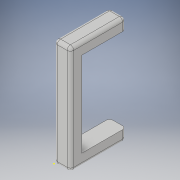
# Autodesk Inventor part: Bumper
Saved by Autodesk Inventor 2018 (Build 220112000, 112)
## iProperties
Created: 2018-01-19
Part Number: Bumper
Material: Generic
Document SubType Name: Modeling
Designer: s-4000369
Density: 1 g/cm^3
Appearance: Default
Author: s-4000369
Autodesk Inventor part; units mm, degrees
ref_plane "YZ Plane" through (0, 0, 0) normal (1, 0, 0) x (0, 1, 0)
ref_plane "XZ Plane" through (0, 0, 0) normal (0, 1, 0) x (-1, 0, 0)
ref_plane "XY Plane" through (0, 0, 0) normal (0, 0, 1) x (1, 0, 0)
sketch "Sketch1" plane through (0, 0, 0) normal (1, 0, 0) x (0, 1, 0)
  point P0 (0, 0)
sketch "Sketch2" plane through (0, 0, 0) normal (1, 0, 0) x (0, 1, 0)
  line L0 (0, 0) -> (0, -431.8)
  line L1 (0, -431.8) -> (88.9, -431.8)
  line L2 (88.9, -431.8) -> (88.9, -88.9)
  line L3 (88.9, -88.9) -> (749.3, -88.9)
  line L4 (749.3, -88.9) -> (749.3, -431.8)
  line L5 (749.3, -431.8) -> (838.2, -431.8)
  line L6 (838.2, -431.8) -> (838.2, 0)
  line L7 (838.2, 0) -> (0, 0)
  dimension "d0" = 660.4
  dimension "d1" = 342.9
  dimension "d2" = 342.9
  dimension "d3" = 88.9
  dimension "d4" = 88.9
  dimension "d5" = 88.9
  constraints: 16 end point, 6 perpendicular, 2 vertical
  measures "d0" distance of L2.end L3.end
  measures "d1" distance of L1.end L2.end
  measures "d2" distance of L3.end L4.end
  measures "d3" distance between parallel lines of L7 L3
  measures "d4" distance between parallel lines of L0 L2
  measures "d5" distance between parallel lines of L4 L6
extrude "Extrusion1" add sketch "Sketch2" along normal blind 127
fillet "Fillet1" radius 25.4 14 edges at (127, 419.1, 0) (0, 419.1, 0) (63.5, 838.2, 0) (127, 838.2, -215.9) (0, 838.2, -215.9) (63.5, 0, 0) (127, 0, -215.9) (127, 44.45, -431.8) (127, 793.75, -431.8) (63.5, 838.2, -431.8) (0, 793.75, -431.8) (0, 0, -215.9) (0, 44.45, -431.8) (63.5, 0, -431.8)
sketch "Sketch7" plane through (0, 88.9, -88.9) normal (0, 0, -1) x (-1, 0, 0)
  line L0 (-127, 0) -> (-127, 660.4) projected
  line L1 (-127, 0) -> (-127, 660.4)
  line L2 (-127, 660.4) -> (-127, 647.7)
  line L3 (-127, -63.5) -> (-127, 723.9) projected
  line L4 (-127, 0) -> (-127, 12.7)
  line L5 (-127, 12.7) -> (-127, 139.7)
  line L6 (-127, 139.7) -> (-127, 266.7)
  line L7 (-127, 266.7) -> (-127, 393.7)
  line L8 (-127, 393.7) -> (-127, 520.7)
  line L9 (-127, 520.7) -> (-127, 647.7)
  line L10 (-127, 330.2) -> (0, 330.2)
  line L11 (-127, 520.7) -> (0, 520.7)
  line L12 (0, 0) -> (0, 660.4) projected
  line L13 (-127, 139.7) -> (0, 139.7)
  line L14 (-127, 139.7) -> (-117.475, 139.7)
  line L15 (-127, 330.2) -> (-117.475, 330.2)
  line L16 (-127, 520.7) -> (-117.475, 520.7)
  line L17 (-117.475, 139.7) -> (-117.475, 165.1)
  line L18 (-117.475, 139.7) -> (-117.475, 114.3)
  line L19 (-117.475, 330.2) -> (-117.475, 304.8)
  line L20 (-117.475, 304.8) -> (-117.475, 355.6)
  line L21 (-117.475, 520.7) -> (-117.475, 495.3)
  line L22 (-117.475, 495.3) -> (-117.475, 546.1)
  circle A0 centre (-117.475, 114.3) radius 2.54
  circle A1 centre (-117.475, 165.1) radius 2.54
  circle A2 centre (-117.475, 304.8) radius 2.54
  circle A3 centre (-117.475, 355.6) radius 2.54
  circle A4 centre (-117.475, 495.3) radius 2.54
  circle A5 centre (-117.475, 546.1) radius 2.54
  line L23 (0, 139.7) -> (-9.525, 139.7)
  line L24 (-9.525, 139.7) -> (-9.525, 114.3)
  line L25 (-9.525, 114.3) -> (-9.525, 165.1)
  line L26 (-9.525, 304.8) -> (-9.525, 330.2)
  line L27 (-9.525, 330.2) -> (-9.525, 355.6)
  line L28 (-9.525, 495.3) -> (-9.525, 520.7)
  line L29 (-9.525, 520.7) -> (-9.525, 546.1)
  circle A6 centre (-9.525, 114.3) radius 2.54
  circle A7 centre (-9.525, 165.1) radius 2.54
  circle A8 centre (-9.525, 304.8) radius 2.54
  circle A9 centre (-9.525, 355.6) radius 2.54
  circle A10 centre (-9.525, 495.3) radius 2.54
  circle A11 centre (-9.525, 546.1) radius 2.54
  point P0 (0, -88.9)
  dimension "d52" = 12.7
  dimension "d53" = 12.7
  dimension "d54" = 127
  dimension "d55" = 127
  dimension "d56" = 127
  dimension "d57" = 127
  dimension "d58" = 9.525
  dimension "d59" = 25.4
  dimension "d60" = 25.4
  dimension "d61" = 25.4
  dimension "d62" = 50.8
  dimension "d63" = 25.4
  dimension "d64" = 50.8
  dimension "d65" = 5.08
  dimension "d66" = 9.525
  constraints: 54 end point, 13 point on line, 12 centre point, 12 coincident, 4 perpendicular, 3 horizontal, 2 collinear, 2 vertical, 1 midpoint, 7 other
  measures "d52" distance of L0.end L2.end
  measures "d53" distance of L0.start L4.end
  measures "d54" distance of L4.end L5.end
  measures "d55" distance of L5.end L6.end
  measures "d56" distance of L6.end L7.end
  measures "d57" distance of L7.end L8.end
  measures "d58" distance of L5.end L14.end
  measures "d59" distance of L14.end L17.end
  measures "d60" distance of L14.end L18.end
  measures "d61" distance of L15.end L19.end
  measures "d62" distance of L19.end L20.end
  measures "d63" distance of L16.end L21.end
  measures "d64" distance of L21.end L22.end
  measures "d65" diameter of A0
  measures "d66" distance of L13.end L23.end
extrude "Extrusion7" cut sketch "Sketch7" against normal blind 25.4 contours A5 | A11 | A6 | A0 | A1 | A7 | A8 | A2 | A3 | A9 | A10 | A4
body "Solid1"
